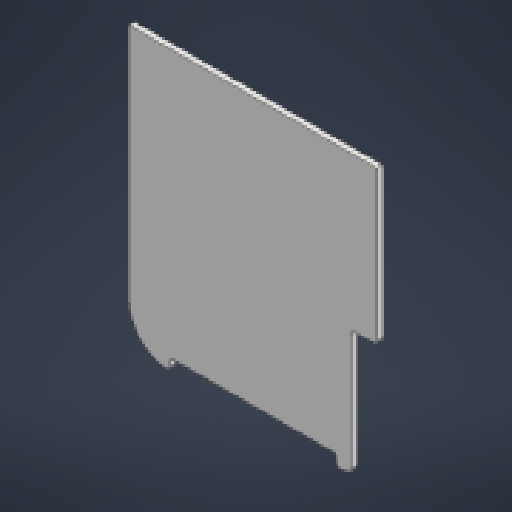
# Autodesk Inventor part: 第二层板
Saved by Autodesk Inventor 2025 (Build 290162000, 162)
## iProperties
Created: 2025-11-17
Part Number: 第二层板
Material: 常规
Document SubType Name: Modeling
Designer: XH
Density: 1 g/cm^3
Appearance: 默认
Author: XH
Autodesk Inventor part; units mm, degrees
ref_plane "YZ Plane" through (0, 0, 0) normal (1, 0, 0) x (0, 1, 0)
ref_plane "XZ Plane" through (0, 0, 0) normal (0, 1, 0) x (-1, 0, 0)
ref_plane "XY Plane" through (0, 0, 0) normal (0, 0, 1) x (1, 0, 0)
sketch "草图1" plane through (0, 0, 0) normal (0, 0, 1) x (1, 0, 0)
  arc A0 (28.2026, -36.6656) -> (33.2026, -31.6656) centre (28.2026, -31.6656) ccw projected
  line L0 (33.2026, -31.6656) -> (33.2026, 37.3344) projected
  line L1 (33.2026, 37.3344) -> (-32.7974, 37.3344) projected
  line L2 (-32.7974, 37.3344) -> (-32.7974, -31.6656) projected
  arc A1 (-32.7974, -31.6656) -> (-27.7974, -36.6656) centre (-27.7974, -31.6656) ccw projected
  line L3 (-27.7974, -36.6656) -> (28.2026, -36.6656) projected
  point P0 (22.1238, -37.5165)
extrude "拉伸1" add sketch "草图1" along normal blind 1.5
sketch "草图2" plane through (0, 0, 1.5) normal (0, 0, 1) x (1, 0, 0)
  line L0 (-21.8762, -36.6656) -> (22.1238, -36.6656)
  line L1 (22.1238, -36.6656) -> (-21.8762, -36.6656)
  line L2 (-21.8762, -36.6656) -> (-21.8762, -33.6656)
  line L3 (-21.8762, -33.6656) -> (22.1238, -33.6656)
  line L4 (22.1238, -33.6656) -> (22.1238, -36.6656)
  line L5 (-27.7974, -36.6656) -> (28.2026, -36.6656) projected
  point P0 (0, 0)
  point P1 (-21.8762, -36.6656)
  dimension "d3" = 3
  constraints: 10 end point, 2 parallel, 1 collinear, 1 horizontal, 1 perpendicular
  measures "d3" distance of L1.end L2.end
extrude "拉伸2" cut sketch "草图2" against normal blind 2
fillet "圆角1" radius 1 2 edges at (-21.8762, -33.6656, 0.75) (22.1238, -33.6656, 0.75)
sketch "草图3" plane through (0, 0, 1.5) normal (0, 0, 1) x (1, 0, 0)
  line L0 (26.2026, 37.3344) -> (33.1347, 37.3344)
  line L1 (33.2026, 37.4521) -> (33.2026, 5.3344)
  line L2 (33.2026, 5.3344) -> (26.2026, 5.3344)
  line L3 (26.2026, 5.3344) -> (26.2026, 37.3344)
  line L4 (33.2026, -31.6656) -> (33.2026, 37.3344) projected
  line L5 (33.2026, 37.3344) -> (-32.7974, 37.3344) projected
  point P0 (0, 0)
  dimension "d10" = 7
  dimension "d11" = 32
  constraints: 8 end point, 2 collinear, 1 horizontal, 1 parallel, 1 perpendicular
  measures "d10" distance between parallel lines of L1 L3
  measures "d11" distance between parallel lines of L0 L2
extrude "拉伸3" cut sketch "草图3" against normal blind 10
fillet "圆角2" radius 1 1 edges at (26.2026, 5.3344, 0.75)
sketch "草图4" plane through (0, 0, 1.5) normal (0, 0, 1) x (1, 0, 0)
  line L0 (33.2026, 5.3344) -> (27.2026, 5.3344) projected
  arc A0 (26.2026, 6.3344) -> (27.2026, 5.3344) centre (27.2026, 6.3344) ccw projected
  line L1 (26.2026, 6.3344) -> (26.2026, 37.3344) projected
  line L2 (26.2026, 37.3344) -> (-32.7974, 37.3344) projected
  line L3 (-32.7974, 37.3344) -> (-32.7974, -31.6656) projected
  arc A1 (-32.7974, -31.6656) -> (-27.7974, -36.6656) centre (-27.7974, -31.6656) ccw projected
  line L4 (-27.7974, -36.6656) -> (-21.8762, -36.6656) projected
  line L5 (-21.8762, -36.6656) -> (-21.8762, -34.6656) projected
  arc A2 (-20.8762, -33.6656) -> (-21.8762, -34.6656) centre (-20.8762, -34.6656) ccw projected
  line L6 (-20.8762, -33.6656) -> (21.1238, -33.6656) projected
  arc A3 (22.1238, -34.6656) -> (21.1238, -33.6656) centre (21.1238, -34.6656) ccw projected
  line L7 (22.1238, -34.6656) -> (22.1238, -36.6656) projected
  line L8 (22.1238, -36.6656) -> (28.2026, -36.6656) projected
  arc A4 (28.2026, -36.6656) -> (33.2026, -31.6656) centre (28.2026, -31.6656) ccw projected
  line L9 (33.2026, -31.6656) -> (33.2026, 5.3344) projected
  line L10 (-32.0578, 36.5949) -> (25.4631, 36.5949)
  line L11 (25.4631, 36.5949) -> (25.4631, 6.3344)
  arc A5 (25.4631, 6.3344) -> (27.2026, 4.5949) centre (27.2026, 6.3344) ccw
  line L12 (27.2026, 4.5949) -> (32.4631, 4.5949)
  line L13 (32.4631, 4.5949) -> (32.4631, -31.6656)
  arc A6 (28.2026, -35.926) -> (32.4631, -31.6656) centre (28.2026, -31.6656) ccw
  line L14 (28.2026, -35.926) -> (22.8633, -35.926)
  line L15 (22.8633, -35.926) -> (22.8633, -34.6656)
  arc A7 (22.8633, -34.6656) -> (21.1238, -32.926) centre (21.1238, -34.6656) ccw
  line L16 (21.1238, -32.926) -> (-20.8762, -32.926)
  arc A8 (-20.8762, -32.926) -> (-22.6158, -34.6656) centre (-20.8762, -34.6656) ccw
  line L17 (-22.6158, -34.6656) -> (-22.6158, -35.926)
  line L18 (-22.6158, -35.926) -> (-27.7974, -35.926)
  arc A9 (-32.0578, -31.6656) -> (-27.7974, -35.926) centre (-27.7974, -31.6656) ccw
  line L19 (-32.0578, -31.6656) -> (-32.0578, 36.5949)
  point P0 (0, 0)
  constraints: 20 end point, 10 point on circle, 5 centre point, 14 other
extrude "拉伸4" cut sketch "草图4" against normal blind 10
